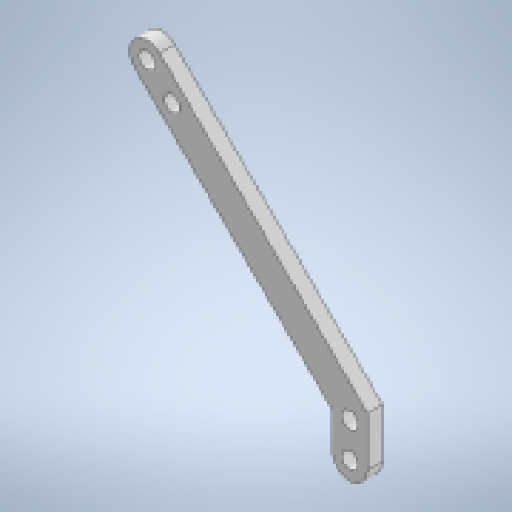
# Autodesk Inventor part: каркас1
Saved by Autodesk Inventor 2023.1 (Build 271208000, 208)
## iProperties
Created: 2025-09-24
Part Number: каркас1
Material: Типовые
Document SubType Name: Modeling
Designer: DELL
Density: 1 g/cm^3
Appearance: По умолчанию
Author: DELL
Autodesk Inventor part; units mm, degrees
ref_plane "YZ Plane" through (0, 0, 0) normal (1, 0, 0) x (0, 1, 0)
ref_plane "XZ Plane" through (0, 0, 0) normal (0, 1, 0) x (-1, 0, 0)
ref_plane "XY Plane" through (0, 0, 0) normal (0, 0, 1) x (1, 0, 0)
sketch "Эскиз1" plane through (0, 0, 0) normal (0, 0, 1) x (1, 0, 0)
  circle A0 centre (-6.3231, 9.8469) radius 1.6
  circle A1 centre (-6.3231, 16.8469) radius 1.6
  line L0 (-6.3231, 9.8469) -> (-6.3231, 16.8469)
  circle A2 centre (-6.3231, 16.8469) radius 3.5
  circle A3 centre (-6.3231, 9.8469) radius 3.5
  line L1 (-9.8231, 9.8469) -> (-9.8231, 16.8469)
  line L2 (-2.8231, 9.8469) -> (-2.8231, 16.8469)
  line L3 (-9.8231, 16.8469) -> (-41.6784, 48.7022)
  line L4 (-9.8231, 16.8469) -> (40.1769, 16.8469) construction
  line L5 (-36.7287, 53.652) -> (-41.6784, 48.7022)
  line L6 (-39.2035, 51.1771) -> (-41.6784, 53.652) construction
  circle A4 centre (-41.6784, 53.652) radius 3.5
  line L7 (-36.7287, 53.652) -> (-2.8231, 19.7464)
  line L8 (-2.8231, 19.7464) -> (-2.8231, 16.8469)
  circle A5 centre (-41.6784, 53.652) radius 1.6
  line L9 (-41.6784, 53.652) -> (-46.6281, 58.6017) construction
  circle A6 centre (-46.6281, 58.6017) radius 3.5
  circle A7 centre (-46.6281, 58.6017) radius 1.6
  line L10 (-41.6784, 48.7022) -> (-49.103, 56.1268)
  line L11 (-36.7287, 53.652) -> (-44.1533, 61.0766)
  point P0 (0, 0)
  dimension "d0" = 3.2
  dimension "d1" = 3.2
  dimension "d2" = 7
  dimension "d3" = 7
  dimension "d4" = 7
  dimension "d8" = 135
  dimension "d9" = 45.0502
  dimension "d10" = 3.5
  dimension "d11" = 7
  dimension "d12" = 3.2
  dimension "d13" = 7
  dimension "d14" = 3.2
  constraints: 24 end point, 7 centre point, 7 coincident, 6 point on circle, 5 tangent, 2 vertical, 1 horizontal, 1 midpoint, 1 perpendicular, 1 point on line, 3 other
  measures "d0" diameter of A0
  measures "d1" diameter of A1
  measures "d2" distance of L0.start L0.end
  measures "d3" diameter of A2
  measures "d4" diameter of A3
  measures "d8" angle of L4 L3
  measures "d9" distance of L1.end L3.end
  measures "d10" distance of L6.start L6.end
  measures "d11" distance from line of L5.start L3
  measures "d12" diameter of A5
  measures "d13" distance of L9.start L9.end
  measures "d14" diameter of A7
extrude "Выдавливание1" add sketch "Эскиз1" along normal blind 3
chamfer "Фаска1" distance 1.5 angle 45 4 edges at (-7.9231, 9.8469, 3) (-7.9231, 16.8469, 3) (-43.2784, 53.652, 3) (-48.2281, 58.6017, 3)
chamfer "Фаска2" distance 1.5 angle 45 4 edges at (-7.9231, 9.8469, 0) (-7.9231, 16.8469, 0) (-43.2784, 53.652, 0) (-48.2281, 58.6017, 0)
